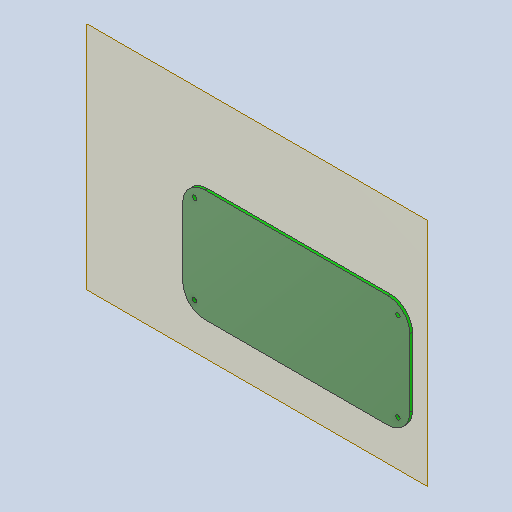
# Autodesk Inventor part: плата
Saved by Autodesk Inventor 2024.2 (Build 282272000, 272)
## iProperties
Created: 2026-02-06
Part Number: плата
Material: Типовые
Document SubType Name: Modeling
Designer: Service
Density: 1 g/cm^3
Appearance: По умолчанию
Author: Service
Autodesk Inventor part; units mm, degrees
ref_plane "YZ Plane" through (0, 0, 0) normal (1, 0, 0) x (0, 1, 0)
ref_plane "XZ Plane" through (0, 0, 0) normal (0, 1, 0) x (-1, 0, 0)
ref_plane "XY Plane" through (0, 0, 0) normal (0, 0, 1) x (1, 0, 0)
ref_plane "РабПлоскость1" through (27.5346, 24.591, 0) normal (0, 0, 1) x (1, 0, 0)
sketch "Эскиз1" plane through (27.5346, 24.591, 0) normal (0, 0, 1) x (1, 0, 0)
  line L0 (90.0933, -53.6999) -> (-33.7344, -53.6999)
  line L1 (-48.7344, -38.6999) -> (-48.7344, 7.3001)
  line L2 (-33.7344, 22.3001) -> (90.0933, 22.3001)
  line L3 (105.0933, 7.3001) -> (105.0933, -38.6999)
  arc A0 (-48.7344, -38.6999) -> (-33.7344, -53.6999) centre (-33.7344, -38.6999) ccw
  arc A1 (90.0933, -53.6999) -> (105.0933, -38.6999) centre (90.0933, -38.6999) ccw
  arc A2 (105.0933, 7.3001) -> (90.0933, 22.3001) centre (90.0933, 7.3001) ccw
  arc A3 (-33.7344, 22.3001) -> (-48.7344, 7.3001) centre (-33.7344, 7.3001) ccw
  circle A4 centre (97.0933, 14.3001) radius 1.5
  circle A5 centre (-40.7344, 14.3001) radius 1.5
  circle A6 centre (-40.7344, -45.6999) radius 1.5
  circle A7 centre (97.0933, -45.6999) radius 1.5
  point P0 (-27.5346, -24.591)
  dimension "d0" = 15
  dimension "d1" = 76
  dimension "d4" = 3
  dimension "d5" = 8
  dimension "d6" = 8
  dimension "d7" = 8
  dimension "d8" = 8
  dimension "d9" = 8
  dimension "d10" = 8
  dimension "d14" = 8
  dimension "d15" = 8
  constraints: 8 centre point, 8 end point, 8 point on circle, 8 tangent, 6 equal radius, 2 parallel, 1 horizontal, 1 perpendicular
  measures "d0" radius of A0
  measures "d1" distance between parallel lines of L0 L2
  measures "d4" diameter of A4
  measures "d5" horizontal distance of L3.start A4.centre
  measures "d6" vertical distance of L2.end A4.centre
  measures "d7" horizontal distance of L1.end A5.centre
  measures "d8" horizontal distance of L1.start A6.centre
  measures "d9" vertical distance of L2.start A5.centre
  measures "d10" vertical distance of L0.end A6.centre
  measures "d14" horizontal distance of L3.end A7.centre
  measures "d15" vertical distance of A7.centre L0.start
extrude "Выдавливание1" add sketch "Эскиз1" along normal blind 1.8
